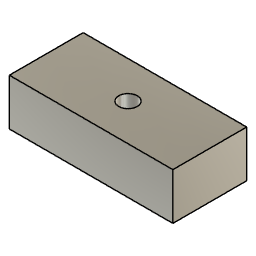
Soporte cámara individual (Parte inferior) (Autodesk Fusion 360 design; units mm, degrees)
Autodesk Fusion 360 part; units mm, degrees
note: some values were not read from the file. Set by a fixed rule: which sketch regions a step uses.
sketch "Boceto1" plane through (0, 0, 0) normal (0, 0, 1) x (1, 0, 0)
  line L0 (24.6, -11.1) -> (-24.6, -11.1)
  line L1 (-24.6, -11.1) -> (-24.6, 11.1)
  line L2 (-24.6, 11.1) -> (24.6, 11.1)
  line L3 (24.6, 11.1) -> (24.6, -11.1)
  line L4 (24.6, -11.1) -> (-24.6, 11.1) construction
  line L5 (-24.6, -11.1) -> (24.6, 11.1) construction
  line L6 (0, 11.1) -> (0, -11.1) construction
  line L7 (-24.6, 0) -> (24.6, 0) construction
  circle A0 centre (0, 0) radius 5.55
  circle A1 centre (0, 0) radius 1.175
  dimension "d9" = 22.2
  dimension "d14" = 11.1
  dimension "d15" = 2.35
  dimension "d34" = 49.2
  constraint horizontal L0
  constraint perpendicular L0 L1
  constraint parallel L0 L2
  constraint parallel L1 L3
  constraint coincident L4 A0.centre
  constraint coincident L5 A0.centre
  constraint coincident A0.centre A1.centre
  constraint midpoint L2 L6.start
  constraint midpoint L0 L6.end
  constraint midpoint L1 L7.start
  constraint midpoint L3 L7.end
  constraint coincident L7 A0.centre
  constraint concentric A0 A1
  measures "d9" distance of L0.end L1.end
  measures "d14" diameter of A0
  measures "d15" diameter of A1
  measures "d34" distance of L1.end L2.end
extrude "Extruir1" add sketch "Boceto1" along normal blind 14 contours L0 L1 L2 L3 | A0 | A1
extrude "Extruir2" cut sketch "Boceto1" along normal blind 2.45 contours A0
extrude "Extruir3" cut sketch "Boceto1" along normal blind 4.9 contours A1
sketch "Boceto2" plane through (0, 0, 14) normal (0, 0, 1) x (-1, 0, 0)
  line L0 (-24.6, -11.1) -> (24.6, -11.1)
  line L1 (24.6, -11.1) -> (24.6, 11.1)
  line L2 (24.6, 11.1) -> (-24.6, 11.1)
  line L3 (-24.6, 11.1) -> (-24.6, -11.1)
  line L4 (24.6, 0) -> (-24.6, 0) construction
  line L5 (0, 11.1) -> (0, -11.1) construction
  circle A0 centre (0, 0) radius 2.8
  dimension "d31" = 5.6
  constraint midpoint L1 L4.start
  constraint midpoint L3 L4.end
  constraint midpoint L2 L5.start
  constraint midpoint L0 L5.end
  constraint coincident L5 A0.centre
  constraint coincident L4 A0.centre
  measures "d31" diameter of A0
extrude "Extruir4" cut sketch "Boceto2" against normal blind 6 contours A0
equation "grosor1 = 2.8 mm"
equation "grosor2 = 2 mm"
equation "grosor3 = 7.5 mm"
equation "tolerancia = 0.1 mm"
equation "diametro_grande_iman = 11 mm"
equation "diametro_pequeno_iman = 2.25 mm"
equation "altura_grande_iman = 2.45 mm"
equation "altura_pequena_iman = 2.45 mm"
equation "d9 = 18 mm + tolerancia * 2 + grosor2 * 2"
equation "DIP_pequena = 41 mm"
equation "DIP_media = 63 mm"
equation "d14 = diametro_grande_iman + tolerancia"
equation "d15 = diametro_pequeno_iman + tolerancia"
equation "grosor4 = 11 mm"
equation "d27 = altura_grande_iman"
equation "d29 = altura_pequena_iman + altura_grande_iman"
equation "d31 = 5.5 mm + tolerancia"
equation "d34 = 45 mm + tolerancia * 2 + grosor2 * 2"
